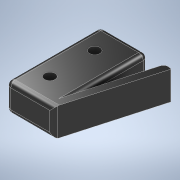
# Autodesk Inventor part: Endstop
Saved by Autodesk Inventor 2021 (Build 250183000, 183)
## iProperties
Created: 2021-04-15
Part Number: Endstop
Material: Generic
Document SubType Name: Modeling
Designer: Fabijan_Sven
Density: 1 g/cm^3
Appearance: Glossy - Black
Author: Fabijan_Sven
Autodesk Inventor part; units mm, degrees
ref_plane "YZ Plane" through (0, 0, 0) normal (1, 0, 0) x (0, 1, 0)
ref_plane "XZ Plane" through (0, 0, 0) normal (0, 1, 0) x (-1, 0, 0)
ref_plane "XY Plane" through (0, 0, 0) normal (0, 0, 1) x (1, 0, 0)
sketch "Sketch1" plane through (0, 0, 0) normal (0, 1, 0) x (-1, 0, 0)
  line L0 (0, 0) -> (10, 0)
  line L1 (10, 0) -> (10, -20)
  line L2 (10, -20) -> (0, -20)
  line L3 (0, -20) -> (0, 0)
  dimension "d0" = 20
  dimension "d1" = 10
  constraints: 8 end point, 2 parallel, 1 horizontal, 1 perpendicular
  measures "d0" distance of L0.end L1.end
  measures "d1" distance of L1.end L2.end
extrude "Extrusion1" add sketch "Sketch1" along normal blind 6
sketch "Sketch2" plane through (0, 6, 0) normal (0, 1, 0) x (1, 0, 0)
  circle A0 centre (-6, 5.25) radius 1.1
  circle A1 centre (-6, 14.75) radius 1.1
  line L0 (-10, 20) -> (-10, 0) projected
  line L1 (0, 20) -> (-10, 20) projected
  point P0 (0, 0)
  dimension "d4" = 2.2
  dimension "d5" = 2.2
  dimension "d6" = 9.5
  dimension "d7" = 4
  dimension "d8" = 4
  dimension "d9" = 5.25
  constraints: 2 centre point
  measures "d4" diameter of A0
  measures "d5" diameter of A1
  measures "d6" distance of A1.centre A0.centre
  measures "d7" distance from line of L0 A0.centre
  measures "d8" distance from line of L0 A1.centre
  measures "d9" distance from line of L1 A1.centre
extrude "Extrusion2" cut sketch "Sketch2" against normal blind 6
sketch "Sketch3" plane through (0, 6, 0) normal (0, 1, 0) x (1, 0, 0)
  line L0 (-1.1092, 1.7066) -> (4.0185, 19.8124)
  line L1 (4.0185, 19.8124) -> (5.4927, 19.3949)
  line L2 (-10, 0) -> (0, 0) projected
  line L3 (5.4927, 19.3949) -> (0, 0)
  line L4 (-1.1092, 1.7066) -> (0, 0)
  constraints: 8 end point, 2 perpendicular
extrude "Extrusion3" add sketch "Sketch3" against normal blind 6
fillet "Fillet1" radius 1 13 edges at (0, 6, -12.8116) (0, 3, -20) (-5, 6, -20) (-5, 0, -20) (-5, 6, 0) (-10, 6, -10) (-10, 3, 0) (-10, 0, -10) (-10, 3, -20) (-5, 0, 0) (0, 3, 0) (0, 0, -12.8116) (4.0185, 3, -19.8124)
body "Solid1"
